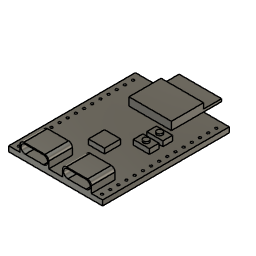
base_station_enclosure_esp32-c3-devkitm-1 v8 (Autodesk Fusion 360 archive; units mm, degrees)
design "esp32-c3-devkitm-1"
Autodesk Fusion 360 part; units mm, degrees
note: some values were not read from the file. Set by a fixed rule: the direction of a hole.
sketch "Sketch1" plane through (0, 0, 0) normal (0, 0, 1) x (1, 0, 0) in component "esp32-c3-devkitm-1"
  line L0 (14.6, 39.4) -> (-14.6, 39.4)
  line L1 (-14.6, 39.4) -> (-14.6, 0)
  line L2 (-14.6, 0) -> (14.6, 0)
  line L3 (14.6, 0) -> (14.6, 39.4)
  line L4 (14.6, 39.4) -> (-14.6, 0) construction
  line L5 (-14.6, 39.4) -> (14.6, 0) construction
  line L6 (0, 1.75) -> (0, 22.5)
  line L7 (1.75, 0) -> (22.5, 0)
  line L8 (6.6, 39.4) -> (-6.6, 39.4)
  line L9 (-6.6, 39.4) -> (-6.6, 29.4)
  line L10 (-6.6, 29.4) -> (6.6, 29.4)
  line L11 (6.6, 29.4) -> (6.6, 39.4)
  line L12 (6.6, 39.4) -> (-6.6, 29.4) construction
  line L13 (-6.6, 39.4) -> (6.6, 29.4) construction
  line L14 (6.6, 45) -> (-6.6, 45)
  line L15 (-6.6, 45) -> (-6.6, 39.4)
  line L16 (-6.6, 39.4) -> (6.6, 39.4)
  line L17 (6.6, 39.4) -> (6.6, 45)
  line L18 (6.6, 45) -> (-6.6, 39.4) construction
  line L19 (-6.6, 45) -> (6.6, 39.4) construction
  line L20 (-2.15, 7.35) -> (-11.1, 7.35)
  line L21 (-11.1, 7.35) -> (-11.1, 0)
  line L22 (-11.1, 0) -> (-2.15, 0)
  line L23 (-2.15, 0) -> (-2.15, 7.35)
  line L24 (-2.15, 7.35) -> (-11.1, 0) construction
  line L25 (-11.1, 7.35) -> (-2.15, 0) construction
  line L26 (11.1, 7.35) -> (2.15, 7.35)
  line L27 (2.15, 7.35) -> (2.15, 0)
  line L28 (2.15, 0) -> (11.1, 0)
  line L29 (11.1, 0) -> (11.1, 7.35)
  line L30 (11.1, 7.35) -> (2.15, 0) construction
  line L31 (2.15, 7.35) -> (11.1, 0) construction
  line L32 (2.5, 17.7) -> (-2.5, 17.7)
  line L33 (-2.5, 17.7) -> (-2.5, 12.7)
  line L34 (-2.5, 12.7) -> (2.5, 12.7)
  line L35 (2.5, 12.7) -> (2.5, 17.7)
  line L36 (2.5, 17.7) -> (-2.5, 12.7) construction
  line L37 (-2.5, 17.7) -> (2.5, 12.7) construction
  line L38 (9.6, 26.75) -> (4.6, 26.75)
  line L39 (4.6, 26.75) -> (4.6, 23.75)
  line L40 (4.6, 23.75) -> (9.6, 23.75)
  line L41 (9.6, 23.75) -> (9.6, 26.75)
  line L42 (9.6, 26.75) -> (4.6, 23.75) construction
  line L43 (4.6, 26.75) -> (9.6, 23.75) construction
  line L44 (9.6, 22.55) -> (4.6, 22.55)
  line L45 (4.6, 22.55) -> (4.6, 19.55)
  line L46 (4.6, 19.55) -> (9.6, 19.55)
  line L47 (9.6, 19.55) -> (9.6, 22.55)
  line L48 (9.6, 22.55) -> (4.6, 19.55) construction
  line L49 (4.6, 22.55) -> (9.6, 19.55) construction
  circle A0 centre (7.1, 25.25) radius 0.9
  circle A1 centre (7.1, 21.05) radius 0.9
  circle A2 centre (12.95, 37.025) radius 0.5
  circle A3 centre (-12.95, 37.025) radius 0.5
  circle A4 centre (12.95, 34.485) radius 0.5
  circle A5 centre (-12.95, 34.485) radius 0.5
  circle A6 centre (12.95, 31.945) radius 0.5
  circle A7 centre (-12.95, 31.945) radius 0.5
  circle A8 centre (12.95, 29.405) radius 0.5
  circle A9 centre (-12.95, 29.405) radius 0.5
  circle A10 centre (12.95, 26.865) radius 0.5
  circle A11 centre (-12.95, 26.865) radius 0.5
  circle A12 centre (12.95, 24.325) radius 0.5
  circle A13 centre (-12.95, 24.325) radius 0.5
  circle A14 centre (12.95, 21.785) radius 0.5
  circle A15 centre (-12.95, 21.785) radius 0.5
  circle A16 centre (12.95, 19.245) radius 0.5
  circle A17 centre (-12.95, 19.245) radius 0.5
  circle A18 centre (12.95, 16.705) radius 0.5
  circle A19 centre (-12.95, 16.705) radius 0.5
  circle A20 centre (12.95, 14.165) radius 0.5
  circle A21 centre (-12.95, 14.165) radius 0.5
  circle A22 centre (12.95, 11.625) radius 0.5
  circle A23 centre (-12.95, 11.625) radius 0.5
  circle A24 centre (12.95, 9.085) radius 0.5
  circle A25 centre (-12.95, 9.085) radius 0.5
  circle A26 centre (12.95, 6.545) radius 0.5
  circle A27 centre (-12.95, 6.545) radius 0.5
  circle A28 centre (12.95, 4.005) radius 0.5
  circle A29 centre (-12.95, 4.005) radius 0.5
  circle A30 centre (12.95, 1.465) radius 0.5
  circle A31 centre (-12.95, 1.465) radius 0.5
  point P0 (0, 19.7)
  point P1 (0, 34.4)
  point P2 (0, 42.2)
  point P3 (-6.625, 3.675)
  point P4 (6.625, 3.675)
  point P5 (0, 15.2)
  point P6 (7.1, 25.25)
  point P7 (7.1, 21.05)
  dimension "d22" = 29.2
  dimension "d23" = 39.4
  dimension "d24" = 13.2
  dimension "d25" = 10
  dimension "d26" = 13.2
  dimension "d27" = 5.6
  dimension "d28" = 8.95
  dimension "d29" = 7.35
  dimension "d31" = 3.5
  dimension "d32" = 8.95
  dimension "d33" = 7.35
  dimension "d34" = 3.5
  dimension "d35" = 5
  dimension "d36" = 5
  dimension "d37" = 17.7
  dimension "d41" = 5
  dimension "d42" = 3
  dimension "d43" = 10
  dimension "d44" = 12.65
  dimension "d45" = 5
  dimension "d46" = 3
  dimension "d47" = 1.2
  dimension "d48" = 1.8
  dimension "d49" = 1.8
  dimension "d95" = 2.375
  dimension "d96" = 1.65
  dimension "d99" = -25.9
  dimension "d105" = 1
  constraint horizontal L0
  constraint perpendicular L0 L1
  constraint parallel L0 L2
  constraint parallel L1 L3
  constraint coincident L4 P0
  constraint coincident L5 P0
  constraint coincident P0 L6
  constraint collinear L2 L7
  constraint horizontal L8
  constraint perpendicular L8 L9
  constraint parallel L8 L10
  constraint parallel L9 L11
  constraint coincident L12 P1
  constraint coincident L13 P1
  constraint coincident L6 P1
  constraint collinear L0 L8
  constraint horizontal L14
  constraint perpendicular L14 L15
  constraint parallel L14 L16
  constraint parallel L15 L17
  constraint coincident L18 P2
  constraint coincident L19 P2
  constraint coincident L6 P2
  constraint collinear L8 L16
  constraint horizontal L20
  constraint perpendicular L20 L21
  constraint parallel L20 L22
  constraint parallel L21 L23
  constraint coincident L24 P3
  constraint coincident L25 P3
  constraint collinear L2 L22
  constraint horizontal L26
  constraint perpendicular L26 L27
  constraint parallel L26 L28
  constraint parallel L27 L29
  constraint coincident L30 P4
  constraint coincident L31 P4
  constraint collinear L2 L28
  constraint horizontal L32
  constraint perpendicular L32 L33
  constraint parallel L32 L34
  constraint parallel L33 L35
  constraint coincident L36 P5
  constraint coincident L37 P5
  constraint coincident L6 P5
  constraint horizontal L38
  constraint perpendicular L38 L39
  constraint parallel L38 L40
  constraint parallel L39 L41
  constraint coincident L42 P6
  constraint coincident L43 P6
  constraint horizontal L44
  constraint perpendicular L44 L45
  constraint parallel L44 L46
  constraint parallel L45 L47
  constraint coincident L48 P7
  constraint coincident L49 P7
  constraint collinear L39 L45
  constraint midpoint L43 P6
  constraint midpoint L49 P7
  measures "d22" distance of L1.end L2.end
  measures "d23" distance of L0.end L1.end
  measures "d24" distance of L9.end L10.end
  measures "d25" distance of L8.end L9.end
  measures "d26" distance of L8.end L8.start
  measures "d27" distance of L14.end L8.end
  measures "d28" distance of L21.end L22.end
  measures "d29" distance of L20.end L21.end
  measures "d31" distance of L1 L21
  measures "d32" distance of L27.end L28.end
  measures "d33" distance of L26.end L27.end
  measures "d34" distance of L3 L29
  measures "d35" distance of L33.end L34.end
  measures "d36" distance of L32.end L33.end
  measures "d37" distance of L2 L32
  measures "d41" distance of L39.end L40.end
  measures "d42" distance of L38.end L39.end
  measures "d43" distance of L3 L39
  measures "d44" distance of L0 L38
  measures "d45" distance of L45.end L46.end
  measures "d46" distance of L44.end L45.end
  measures "d47" distance of L40 L44
  measures "d48" diameter of A0
  measures "d49" diameter of A1
  measures "d95" distance of L0 A2.centre
  measures "d96" distance of L3 A2.centre
  measures "d105" diameter of A2
extrude "Extrude1" add sketch "Sketch1" along normal blind 1.6 contours L0 L1 L2 L3 L7 L9 L10 L11 L20 L21 L23 L26 L27 L29 | A2 | A3 | A4 | A5 | A6 | A7 | A8 | A9 | A10 | A11 | A12 | A13 | A14 | A15 | A16 | A17 | A18 | A19 | A20 | A21 | A22 | A23 | A24 | A25 | A26 | A27 | A28 | A29 | A30 | A31 in component "esp32-c3-devkitm-1"
extrude "Extrude2" add sketch "Sketch1" along normal blind 4.9 contours L2 L7 L26 L27 L28 L29 | L2 L20 L21 L22 L23 in component "esp32-c3-devkitm-1"
extrude "Extrude3" add sketch "Sketch1" along normal blind 4.1 contours L0 L8 L9 L10 L11 L16 in component "esp32-c3-devkitm-1"
extrude "Extrude4" add sketch "Sketch1" along normal blind 3.15 contours L6 L32 L33 L34 | L6 L32 L34 L35 in component "esp32-c3-devkitm-1"
extrude "Extrude5" add sketch "Sketch1" along normal blind 3.15 contours L38 L39 L40 L41 | L44 L45 L46 L47 in component "esp32-c3-devkitm-1"
extrude "Extrude6" add sketch "Sketch1" along normal blind 3.65 contours A0 | A1 in component "esp32-c3-devkitm-1"
extrude "Extrude7" add sketch "Sketch1" along normal blind 0.8 from surface at 1.6 contours L0 L8 L14 L15 L16 L17 in component "esp32-c3-devkitm-1"
fillet "Fillet1" radius 1.2 4 edges at (-11.1, 3.675, 4.9) (-2.15, 3.675, 4.9) (2.15, 3.675, 4.9) (11.1, 3.675, 4.9) in component "esp32-c3-devkitm-1"
sketch "Sketch2" plane through (0, 0, 0) normal (0, -1, 0) x (1, 0, 0) in component "esp32-c3-devkitm-1"
  arc A0 (11.1, 3.7) -> (9.9, 4.9) centre (9.9, 3.7) ccw
  line L0 (9.9, 4.9) -> (3.35, 4.9)
  arc A1 (3.35, 4.9) -> (2.15, 3.7) centre (3.35, 3.7) ccw
  line L1 (2.15, 3.7) -> (2.15, 1.6)
  line L2 (2.15, 1.6) -> (-2.15, 1.6)
  line L3 (-2.15, 1.6) -> (-2.15, 3.7)
  arc A2 (-2.15, 3.7) -> (-3.35, 4.9) centre (-3.35, 3.7) ccw
  line L4 (-3.35, 4.9) -> (-9.9, 4.9)
  arc A3 (-9.9, 4.9) -> (-11.1, 3.7) centre (-9.9, 3.7) ccw
  line L5 (-11.1, 3.7) -> (-11.1, 1.6)
  line L6 (-11.1, 1.6) -> (-14.6, 1.6)
  line L7 (-14.6, 1.6) -> (-14.6, 0)
  line L8 (-14.6, 0) -> (14.6, 0)
  line L9 (14.6, 0) -> (14.6, 1.6)
  line L10 (14.6, 1.6) -> (11.1, 1.6)
  line L11 (11.1, 1.6) -> (11.1, 3.7)
  line L12 (-9.45, 4.6) -> (-3.8, 4.6)
  line L13 (-9.45, 1.9) -> (-3.8, 1.9)
  arc A4 (-9.45, 4.6) -> (-9.45, 1.9) centre (-9.45, 3.25) ccw
  arc A5 (-3.8, 1.9) -> (-3.8, 4.6) centre (-3.8, 3.25) ccw
  arc A6 (9.45, 1.9) -> (9.45, 4.6) centre (9.45, 3.25) ccw
  line L14 (3.8, 1.9) -> (9.45, 1.9)
  arc A7 (3.8, 4.6) -> (3.8, 1.9) centre (3.8, 3.25) ccw
  line L15 (3.8, 4.6) -> (9.45, 4.6)
  dimension "d80" = 0.3
  dimension "d81" = 1.65
  dimension "d83" = 0.3
  dimension "d86" = 0.3
  dimension "d87" = 1.65
  dimension "d88" = 1.65
  dimension "d89" = 1.65
  dimension "d90" = 1.65
  dimension "d91" = 0.3
  dimension "d92" = 1.65
  dimension "d93" = 1.65
  dimension "d94" = 1.65
  constraint parallel L4 L12
  constraint tangent L13 A4
  constraint tangent L13 A5
  constraint tangent L14 A7
  constraint tangent A6 L14
  measures "d80" distance of L4 L12
  measures "d81" distance of L5 L12.start
  measures "d83" distance of L6 L13
  measures "d86" distance of L0 L15
  measures "d87" distance of L11 A6.end
  measures "d88" distance of L11 A6.start
  measures "d89" distance of L1 L14.start
  measures "d90" distance of L1 A7.start
  measures "d91" distance of L10 L14
  measures "d92" distance of L3 L12.end
  measures "d93" distance of L3 L13.end
  measures "d94" distance of L5 L13.start
extrude "Extrude8" cut sketch "Sketch2" against normal blind 7 contours L12 L13 A4 A5 | A6 L14 A7 L15 in component "esp32-c3-devkitm-1"
hole "Hole2" at (12.95, 37.025, 0) at (12.95, 34.485, 0) at (12.95, 31.945, 0) at (12.95, 29.405, 0) at (12.95, 26.865, 0) at (12.95, 24.325, 0) at (12.95, 21.785, 0) at (12.95, 19.245, 0) at (12.95, 16.705, 0) at (12.95, 14.165, 0) at (12.95, 11.625, 0) at (12.95, 9.085, 0) at (12.95, 6.545, 0) at (12.95, 4.005, 0) at (12.95, 1.465, 0) at (-12.95, 1.465, 0) at (-12.95, 4.005, 0) at (-12.95, 6.545, 0) at (-12.95, 9.085, 0) at (-12.95, 11.625, 0) at (-12.95, 14.165, 0) at (-12.95, 16.705, 0) at (-12.95, 19.245, 0) at (-12.95, 21.785, 0) at (-12.95, 24.325, 0) at (-12.95, 26.865, 0) at (-12.95, 29.405, 0) at (-12.95, 31.945, 0) at (-12.95, 34.485, 0) at (-12.95, 37.025, 0) direction (0, 0, 1) diameter 0.75 depth 11 tip angle 118 in component "esp32-c3-devkitm-1"
component "esp32-c3-devkitm-1" placed x (1, 0, 0) y (0, 1, 0) z (0, 0, 1) at (0, 0, 0)
equation "pcb_thickness = 1.6 mm"
equation "module_height = 2.5 mm"
equation "usb_height = 3.3 mm"
equation "button_modue_height = 1.55 mm"
equation "button_height = 0.5 mm"
equation "button_diameter = 1.8 mm"
equation "led_height = 1.55 mm"
equation "pin_count = 15"
equation "led_width_length = 5 mm"
equation "usb_width = 8.95 mm"
equation "usb_length = 7.35 mm"
equation "board_length = 39.4 mm"
equation "board_width = 29.2 mm"
equation "overall_length = 45 mm"
equation "module_width = 13.2 mm"
equation "module_length = 10 mm"
equation "button_module_width = 3 mm"
equation "button_module_length = 5 mm"
equation "pin_spacing = 2.54 mm"
equation "d22 = board_width"
equation "d23 = board_length"
equation "d24 = module_width"
equation "d25 = module_length"
equation "d26 = module_width"
equation "d27 = overall_length - board_length"
equation "d28 = usb_width"
equation "d29 = usb_length"
equation "d32 = usb_width"
equation "d33 = usb_length"
equation "d35 = led_width_length"
equation "d36 = led_width_length"
equation "d41 = button_module_length"
equation "d42 = button_module_width"
equation "d44 = 15.65 mm - button_module_width"
equation "d45 = button_module_length"
equation "d46 = button_module_width"
equation "d48 = button_diameter"
equation "d49 = button_diameter"
equation "d50 = pcb_thickness"
equation "d52 = pcb_thickness + usb_height"
equation "d54 = pcb_thickness + module_height"
equation "d56 = pcb_thickness + led_height"
equation "d58 = pcb_thickness + button_modue_height"
equation "d60 = pcb_thickness + button_modue_height + button_height"
equation "d62 = pcb_thickness"
equation "d98 = pin_count"
equation "d99 = -( board_width - 1.65 mm - 1.65 mm )"
equation "d100 = -pin_spacing"
equation "pin_diameter = 1 mm"
equation "d105 = pin_diameter"
equation "tolerance_loose = 0.508 mm"
equation "tolerance_tight = 0.127 mm"
equation "tolerance_normal = 0.254 mm"
equation "sma_base_plate_widthy = 6.55 mm"
equation "antenna_board_thickness = 3.225 mm"
equation "sma_base_plate_thickness = 1.65 mm"
equation "antenna_header_width_offset = 5.25 mm"
equation "antenna_header_length_offset = 1.3 mm"
equation "sma_base_plate_vertical_offset = 1 mm"
equation "antenna_board_length_Copy = 33.3 mm"
equation "antenna_board_width = 18 mm"
equation "sma_width_offset = 9 mm"
equation "sma_diameter = 6.26 mm"
equation "antenna_sma_wall_thickness = 3.15 mm"
